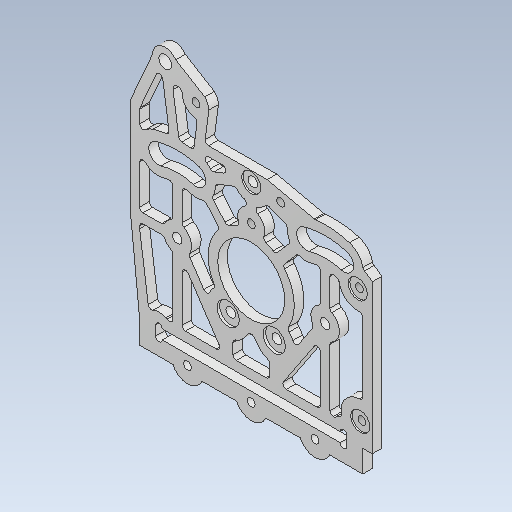
# Autodesk Inventor part: 中間フレーム内側
Saved by Autodesk Inventor 2020.2 (Build 242310000, 310)
## iProperties
Created: 2020-03-13
Part Number: 中間フレーム内側
Material: アルミニウム 2014-T4
Document SubType Name: Modeling
Designer: aoyam
Density: 2.8 g/cm^3
Appearance: サテン
Mass: 22.5667 g
Surface Area: 94.6631 cm^2
Volume: 8.05954 cm^3
Author: aoyam
Autodesk Inventor part; units mm, degrees
ref_plane "YZ Plane" through (0, 0, 0) normal (1, 0, 0) x (0, 1, 0)
ref_plane "XZ Plane" through (0, 0, 0) normal (0, 1, 0) x (-1, 0, 0)
ref_plane "XY Plane" through (0, 0, 0) normal (0, 0, 1) x (1, 0, 0)
sketch "スケッチ1" plane through (0, 0, 0) normal (0, 0, 1) x (1, 0, 0)
  circle A0 centre (0, 15.5) radius 1.25
  circle A1 centre (0, -15.5) radius 1.5
  line L0 (0, 0) -> (100, 0)
  line L1 (0, 15.5) -> (0, -15.5)
  circle A2 centre (23.2, 20.8573) radius 1.5
  circle A3 centre (23.2, 0) radius 1.5
  line L2 (23.2, 20.8573) -> (23.2, 0)
  line L3 (23.2, 0) -> (90.6993, -20)
  line L4 (23.2, 0) -> (29.1254, 19.9979)
  line L5 (23.2, 0) -> (17.2746, 19.9979)
  arc A4 (29.1254, 19.9979) -> (17.2746, 19.9979) centre (23.2, 0) ccw construction
  arc A5 (29.9847, 22.8983) -> (16.4153, 22.8983) centre (23.2, 0) ccw
  arc A6 (28.266, 17.0975) -> (18.134, 17.0975) centre (23.2, 0) ccw
  arc A7 (28.266, 17.0975) -> (29.9847, 22.8983) centre (29.1254, 19.9979) ccw
  arc A8 (16.4153, 22.8983) -> (18.134, 17.0975) centre (17.2746, 19.9979) ccw
  circle A9 centre (0, 0) radius 10.5
  circle A10 centre (0, 0) radius 14.1421
  circle A11 centre (0, 15.5) radius 4.5
  circle A12 centre (0, -15.5) radius 4.5
  line L6 (0, 30) -> (38, 30)
  line L7 (38, 30) -> (38, -28)
  line L8 (38, -28) -> (0, -28)
  line L9 (0, -28) -> (0, 30)
  circle A13 centre (-23.2, 0) radius 1.5
  arc A14 (-16.4153, 22.8983) -> (-29.9847, 22.8983) centre (-23.2, 0) ccw
  arc A15 (-18.134, 17.0975) -> (-28.266, 17.0975) centre (-23.2, 0) ccw
  arc A16 (-29.9847, 22.8983) -> (-28.266, 17.0975) centre (-29.1254, 19.9979) ccw
  arc A17 (-18.134, 17.0975) -> (-16.4153, 22.8983) centre (-17.2746, 19.9979) ccw
  line L10 (0, 30) -> (-38, 30)
  line L11 (-38, 30) -> (-38, -28)
  line L12 (-38, -28) -> (0, -28)
  line L13 (-38, -27) -> (38, -27)
  line L14 (-30, -27) -> (30, -27)
  line L15 (30, -27) -> (30, -30)
  line L16 (30, -30) -> (-30, -30)
  line L17 (-30, -30) -> (-30, -27)
  line L18 (0, -27) -> (0, -33)
  circle A18 centre (0, -33) radius 1.25
  circle A19 centre (-20, -33) radius 1.25
  circle A20 centre (20, -33) radius 1.25
  circle A21 centre (-20, -33) radius 5
  circle A22 centre (0, -33) radius 5
  circle A23 centre (20, -33) radius 5
  line L19 (35, -22) -> (-35, -22)
  line L20 (-35, -22) -> (-35, -35)
  line L21 (-35, -35) -> (35, -35)
  line L22 (35, -35) -> (35, -22)
  circle A24 centre (-28.95, -27) radius 1.05
  line L23 (-30, -27) -> (-28.95, -27)
  line L24 (-12.3917, -28.5) -> (-10.5848, -28.5)
  circle A25 centre (-28.95, -30) radius 1.05
  circle A26 centre (28.95, -27) radius 1.05
  circle A27 centre (28.95, -30) radius 1.05
  line L25 (30, -27) -> (30, -30)
  line L26 (-30, -27) -> (-30, -30)
  circle A28 centre (-27, 46) radius 2
  circle A29 centre (-27, 46) radius 4
  line L27 (-38, 30) -> (-31, 46)
  line L28 (-23.4377, 47.8194) -> (-19, 30)
  circle A30 centre (-17.3043, 39.7432) radius 4
  circle A31 centre (-17.3043, 39.7432) radius 1.25
  line L29 (-23.6785, 48.2289) -> (-14.5834, 42.6752)
  line L30 (-13.3043, 39.7432) -> (-14.5834, 30)
  line L31 (27.4137, -1.5794) -> (34.5946, 17.4704)
  arc A32 (34.5946, 17.4704) -> (30.837, 25.7747) centre (29.1254, 19.9979) ccw
  arc A33 (30.837, 25.7747) -> (23.2, 26.8823) centre (23.2, 0) ccw
  line L32 (23.2, 26.8823) -> (-8.2253, 30.1221)
  arc A34 (-8.2253, 30.1221) -> (-10.295, 30.1221) centre (-9.2601, 26) ccw
  line L33 (-10.295, 30.1221) -> (-23.2, 26.8823)
  arc A35 (-23.2, 26.8823) -> (-30.837, 25.7747) centre (-23.2, 0) ccw
  arc A36 (-30.837, 25.7747) -> (-34.7286, 17.7833) centre (-29.1254, 19.9979) ccw
  line L34 (-34.7286, 17.7833) -> (-27.7, 0)
  arc A37 (-27.7, 0) -> (-25.9762, -3.5416) centre (-23.2, 0) ccw
  line L35 (-25.9762, -3.5416) -> (-10.0045, -16.0614)
  arc A38 (-10.0045, -16.0614) -> (-7.2283, -17.0198) centre (-7.2283, -12.5198) ccw
  line L36 (-7.2283, -17.0198) -> (7.2283, -17.0198)
  arc A39 (7.2283, -17.0198) -> (10.0045, -16.0614) centre (7.2283, -12.5198) ccw
  line L37 (10.0045, -16.0614) -> (25.9762, -3.5416)
  arc A40 (25.9762, -3.5416) -> (27.4137, -1.5794) centre (23.2, 0) ccw
  circle A41 centre (-7.2283, -12.5198) radius 1.5
  circle A42 centre (23.2, 0) radius 1.5
  circle A43 centre (-23.2, 0) radius 1.5
  circle A44 centre (7.2283, -12.5198) radius 1.5
  circle A45 centre (-9.2601, 26) radius 1.25
  arc A46 (28.266, 17.0975) -> (29.9847, 22.8983) centre (29.1254, 19.9979) ccw
  arc A47 (28.266, 17.0975) -> (18.134, 17.0975) centre (23.2, 0) ccw
  arc A48 (16.4153, 22.8983) -> (18.134, 17.0975) centre (17.2746, 19.9979) ccw
  arc A49 (29.9847, 22.8983) -> (16.4153, 22.8983) centre (23.2, 0) ccw
  arc A50 (-29.9847, 22.8983) -> (-28.266, 17.0975) centre (-29.1254, 19.9979) ccw
  arc A51 (-16.4153, 22.8983) -> (-29.9847, 22.8983) centre (-23.2, 0) ccw
  arc A52 (-18.134, 17.0975) -> (-16.4153, 22.8983) centre (-17.2746, 19.9979) ccw
  arc A53 (-18.134, 17.0975) -> (-28.266, 17.0975) centre (-23.2, 0) ccw
  circle A54 centre (9.2601, 26) radius 1.25
  point P0 (0, 0)
  point P1 (24.7, 0)
  point P2 (38, 0)
  point P3 (38, -4.3852)
  point P4 (24.6382, -0.4261)
  point P5 (0.6086, 14.129)
  point P6 (-0.6086, 14.129)
  point P7 (30, -27)
  point P8 (-35, -28)
  point P9 (-24.5826, -35)
  point P10 (-15.4174, -35)
  point P11 (-4.5826, -35)
  point P12 (4.5826, -35)
  point P13 (15.4174, -35)
  point P14 (24.5826, -35)
  point P15 (35, -28)
  point P16 (-27.9, -30)
  point P17 (-30, -30)
  point P18 (-30, -28.4849)
  point P19 (-27.9, -27)
  point P20 (27.9, -27)
  point P21 (30, -27)
  point P22 (30, -30)
  point P23 (27.9, -30)
  point P24 (-30, -30)
  point P25 (-30, -28)
  point P26 (-29.2702, -28)
  point P27 (29.2702, -28)
  point P28 (30, -28)
  point P29 (29.9846, -28.5)
  point P30 (28.5305, -28.5)
  point P31 (-29.9846, -28.5)
  point P32 (-28.5305, -28.5)
  point P33 (0, -30)
  point P34 (0, -28)
  point P35 (0, -27)
  point P36 (-27.9, -27)
  point P37 (-30, -30)
  point P38 (0, -27)
  point P39 (30, -28)
  point P40 (28.6298, -28)
  point P41 (27.9, -27)
  point P42 (0, -28)
  point P43 (30, -27)
  point P44 (15, 30)
  point P45 (-23.0005, 46.0638)
  dimension "d90" = 2.1
  dimension "d0" = 100
  dimension "d1" = 15.5
  dimension "d2" = 15.5
  dimension "d3" = 3
  dimension "d4" = 2.5
  dimension "d5" = 31
  dimension "d10" = 23.2
  dimension "d12" = 20.8573
  dimension "d13" = 70.4
  dimension "d14" = 90
  dimension "d15" = 20.8573
  dimension "d16" = 20
  dimension "d17" = 6.05
  dimension "d18" = 3
  dimension "d24" = 21
  dimension "d27" = 3.6421
  dimension "d28" = 30
  dimension "d29" = 28
  dimension "d30" = 38
  dimension "d70" = 1
  dimension "d71" = 60
  dimension "d72" = 3
  dimension "d73" = 30
  dimension "d76" = 6
  dimension "d77" = 2.5
  dimension "d80" = 20
  dimension "d85" = 10
  dimension "d86" = 10
  dimension "d87" = 10
  dimension "d88" = 5
  dimension "d93" = 1.5
  dimension "d97" = 4
  dimension "d98" = 8
  dimension "d102" = 8
  dimension "d103" = 2.5
  dimension "d262" = 73
  dimension "d264" = 3
  constraints: 76 end point, 58 point on circle, 52 centre point, 18 symmetric about line, 7 coincident, 7 point on line, 7 vertical, 6 horizontal, 6 parallel, 5 tangent, 4 perpendicular, 3 midpoint, 26 other
  measures "d0" distance of L0.start L0.end
  measures "d1" distance of L1.start L0.start
  measures "d2" distance of L1.end L0.start
  measures "d3" diameter of A1
  measures "d4" diameter of A0
  measures "d5" distance of L1.start L1.end
  measures "d10" distance of L0.start L2.end
  measures "d12" distance of L2.start L2.end
  measures "d13" distance of L2.end L3.end
  measures "d14" angle of L3 L4
  measures "d15" distance of L2.end L4.end
  measures "d16" distance from line of L0 L3.end
  measures "d17" diameter of A8
  measures "d18" diameter of A3
  measures "d24" diameter of A9
  measures "d27" radial gap between concentric circles of A9 A10
  measures "d28" distance from line of L6.end L0
  measures "d29" distance from line of L7.end L0
  measures "d30" distance between parallel lines of L9 L7
  measures "d70" distance between parallel lines of L8 L13
  measures "d71" distance of L15.end L16.end
  measures "d72" distance of L14.end L15.end
  measures "d73" distance between parallel lines of L9 L15
  measures "d76" distance of L18.start L18.end
  measures "d77" diameter of A18
  measures "d80" distance of A18.centre A19.centre
  measures "d85" diameter of A21
  measures "d86" diameter of A22
  measures "d87" diameter of A23
  measures "d88" distance between parallel lines of L13 L19
  measures "d93" distance between parallel lines of L24 L14
  measures "d97" diameter of A28
  measures "d98" diameter of A29
  measures "d102" diameter of A30
  measures "d103" diameter of A31
  measures "d262" distance from line of L14 A28.centre
  measures "d264" distance from line of L17 A28.centre
extrude "押し出し1" add sketch "スケッチ1" along normal blind 3 contours A0 L9 A11 A10 L1 | A0 L1 A10 A11 L9 | L9 L32 A33 A32 L31 L0 A3 L4 A7 A5 A8 L5 A10 A11 | A11 A10 A41 A12 L36 A38 L35 A37 L34 A36 A35 L33 L10 L32 L9 | A10 A11 L1 | L1 A11 A10 | A11 L1 A9 A12 A10 A41 | L32 L10 L9 | L9 L6 L7 L0 L31 A32 A33 L32 | A11 A10 L0 A9 L1 | A41 A10 | A10 A41 | A10 A44 A12 L1 A9 L0 | L0 A3 L3 L31 A40 L37 A39 L36 A12 A10 A44 | L33 A35 A36 L34 A37 L35 A38 L36 A12 L9 L19 L20 L13 L11 L10 | A44 A10 | A10 A44 | A12 L1 A1 A10 | A10 A1 L9 L36 A12 | L7 L3 L31 L0 | L10 L28 A30 L30 | A12 A10 A1 L1 | L5 A6 L2 A3 | A3 L0 L31 L3 | A10 L1 L9 A1 | A1 L1 A10 | L36 L9 A12 | L7 L13 L22 L19 L9 A12 L36 A39 L37 A40 L31 L3 | L10 L27 A29 L28 | A30 L29 L30 | A1 A10 L1 | A12 L36 L9 A1 A10 | L2 A6 L4 A3 | L9 L1 A10 A1 | L9 L36 A12 | L7 L8 L22 L13 | L28 A29 L29 A30 | L19 L22 L13 A26 L9 | L9 L13 A24 L20 L19 | L22 L8 L15 L13 | L13 L20 L12 L11 | A29 L28 | L28 A29 | L22 L21 A23 L16 A27 L15 L8 | L13 L17 L12 L20 | L12 L17 A25 L16 A21 L21 L20 | L16 A22 L21 | L16 A23 L21 A22 | A22 L21 A21 L16 | L21 A23 L16 | A23 L21 | A21 L21 L16 | L21 A22 | L21 A21 | A45
sketch "スケッチ8" plane through (0, 0, 3) normal (0, 0, 1) x (1, 0, 0)
  line L0 (0, 0) -> (0, 13.1)
  line L1 (26.2, 7.3075) -> (26.2, 0)
  line L2 (-139.7061, -70) -> (112.711, -70)
  line L3 (-139.7061, -20) -> (112.711, -20)
  line L4 (-139.7231, -25) -> (112.694, -25)
  circle A0 centre (0, 0) radius 20.05
  circle A1 centre (14.8447, 16.629) radius 2.05
  circle A2 centre (14.8447, 16.629) radius 14
  circle A3 centre (19.3878, -11) radius 2.05
  circle A4 centre (19.3878, -11) radius 14
  circle A5 centre (0, 0) radius 9.1
  line L5 (0, 0) -> (-93.6, 0)
  circle A6 centre (-93.6, 0) radius 25.1
  circle A7 centre (-52.6656, -10.2575) radius 17.1
  circle A8 centre (-23.2, 0) radius 14.1
  circle A9 centre (23.2, 0) radius 14.1
  circle A10 centre (52.6656, -10.2575) radius 17.1
  line L6 (0, 0) -> (93.6, 0)
  circle A11 centre (93.6, 0) radius 25.1
  dimension "d53" = 7.3075
  dimension "d54" = 70
  dimension "d55" = 50
  dimension "d56" = 45
  dimension "d57" = 4.1
  dimension "d58" = 28
  dimension "d59" = 4.1
  dimension "d60" = 28
  dimension "d61" = 22.291
  dimension "d62" = 22.291
  dimension "d63" = 40.1
  dimension "d64" = 18.2
  dimension "d65" = 93.6
  dimension "d66" = 50.2
  dimension "d67" = 34.2
  dimension "d68" = 28.2
  dimension "d69" = 70.4
  constraints: 14 end point, 12 centre point, 7 coincident, 5 tangent, 4 symmetric about line, 3 horizontal, 3 point on line, 2 parallel, 1 vertical, 3 other
  measures "d53" distance of L1.start L1.end
  measures "d54" distance from line of L2 point (0, 0)
  measures "d55" distance between parallel lines of L2 L3
  measures "d56" distance between parallel lines of L2 L4
  measures "d57" diameter of A1
  measures "d58" diameter of A2
  measures "d59" diameter of A3
  measures "d60" diameter of A4
  measures "d61" distance of A1.centre point (0, 0)
  measures "d62" distance of A3.centre point (0, 0)
  measures "d63" diameter of A0
  measures "d64" diameter of A5
  measures "d65" distance of L0.start L5.end
  measures "d66" diameter of A6
  measures "d67" diameter of A7
  measures "d68" diameter of A8
  measures "d69" distance of L5.end A8.centre
sketch "スケッチ3" plane through (0, 0, 0) normal (0, 0, -1) x (-1, 0, 0)
  arc A0 (1.6057, 5.7812) -> (-1.6057, 5.7812) centre (0, 0) ccw
  line L0 (-1.5, -5.8095) -> (-1.5, -12.9019)
  arc A1 (-1.5, -12.9019) -> (1.5, -12.9019) centre (0, -15.5) ccw
  line L1 (1.5, -12.9019) -> (1.5, -5.8095)
  arc A2 (1.5, -5.8095) -> (4.2038, 4.2812) centre (0, 0) ccw
  circle A3 centre (0, -15.5) radius 1.5
  circle A4 centre (0, 0) radius 4
  arc A5 (-4.2038, 4.2812) -> (-1.5, -5.8095) centre (0, 0) ccw
  line L2 (4.2038, 4.2812) -> (6.406, 8.0955)
  circle A6 centre (7.2283, 12.5198) radius 3
  line L3 (3.8079, 9.5955) -> (1.6057, 5.7812)
  line L4 (-1.6057, 5.7812) -> (-3.8079, 9.5955)
  circle A7 centre (-7.2283, 12.5198) radius 3
  line L5 (-6.406, 8.0955) -> (-4.2038, 4.2812)
  arc A8 (6.406, 8.0955) -> (3.8079, 9.5955) centre (7.2283, 12.5198) ccw
  arc A9 (-3.8079, 9.5955) -> (-6.406, 8.0955) centre (-7.2283, 12.5198) ccw
  line L6 (0, 0) -> (-9.4783, 0)
  circle A10 centre (7.2283, -12.5198) radius 3
  circle A11 centre (-7.2283, -12.5198) radius 3
  circle A12 centre (-7.2283, -12.5198) radius 1.5
  circle A13 centre (7.2283, -12.5198) radius 1.5
  point P0 (0, 0)
  point P1 (0, 0)
  dimension "d36" = 3
  dimension "d37" = 3
  constraints: 14 centre point, 14 end point, 12 point on circle, 2 coincident, 2 symmetric about line, 1 horizontal, 4 other
  measures "d36" diameter of A12
  measures "d37" diameter of A13
extrude "押し出し3" cut sketch "スケッチ3" against normal blind 10 contours A12 | A13
sketch "スケッチ2" plane through (0, 0, 3) normal (0, 0, 1) x (1, 0, 0)
  circle A0 centre (0, 15.5) radius 1.25 projected
  circle A1 centre (0, 15.5) radius 3.5
  circle A2 centre (7.2283, -12.5198) radius 1.5 projected
  circle A3 centre (-7.2283, -12.5198) radius 1.5 projected
  circle A4 centre (-7.2283, -12.5198) radius 3.5
  circle A5 centre (7.2283, -12.5198) radius 3.5
  point P0 (0, 0)
  dimension "d33" = 7
  dimension "d40" = 7
  dimension "d41" = 7
  constraints: 3 centre point, 3 coincident
  measures "d33" diameter of A1
  measures "d40" diameter of A4
  measures "d41" diameter of A5
extrude "押し出し2" cut sketch "スケッチ2" against normal blind 0.8 contours A4 | A5
sketch "スケッチ4" plane through (0, 0, 0) normal (0, 0, -1) x (-1, 0, 0)
  circle A0 centre (7.2283, -12.5198) radius 1.5 projected
  circle A1 centre (-7.2283, -12.5198) radius 1.5 projected
  circle A2 centre (-23.2, 0) radius 1.5 projected
  arc A3 (-18.134, 17.0975) -> (-28.266, 17.0975) centre (-23.2, 0) ccw projected
  arc A4 (-29.9847, 22.8983) -> (-28.266, 17.0975) centre (-29.1254, 19.9979) ccw projected
  arc A5 (-16.4153, 22.8983) -> (-29.9847, 22.8983) centre (-23.2, 0) ccw projected
  arc A6 (-18.134, 17.0975) -> (-16.4153, 22.8983) centre (-17.2746, 19.9979) ccw projected
  circle A7 centre (0, 15.5) radius 1.25 projected
  circle A8 centre (0, 0) radius 10.5 projected
  circle A9 centre (23.2, 0) radius 1.5 projected
  arc A10 (28.266, 17.0975) -> (18.134, 17.0975) centre (23.2, 0) ccw projected
  arc A11 (16.4153, 22.8983) -> (18.134, 17.0975) centre (17.2746, 19.9979) ccw projected
  arc A12 (29.9847, 22.8983) -> (16.4153, 22.8983) centre (23.2, 0) ccw projected
  arc A13 (28.266, 17.0975) -> (29.9847, 22.8983) centre (29.1254, 19.9979) ccw projected
  line L0 (-38, -28) -> (-38, 30) projected
  line L1 (-35, -28) -> (-38, -28) projected
  line L2 (38, 30) -> (38, -28) projected
  line L3 (-38, 30) -> (14.5834, 30) projected
  line L4 (-35, -35) -> (-35, -28) projected
  line L5 (-24.5826, -35) -> (-35, -35) projected
  arc A14 (-24.5826, -35) -> (-15.4174, -35) centre (-20, -33) ccw projected
  line L6 (-4.5826, -35) -> (-15.4174, -35) projected
  arc A15 (-4.5826, -35) -> (4.5826, -35) centre (0, -33) ccw projected
  line L7 (15.4174, -35) -> (4.5826, -35) projected
  arc A16 (15.4174, -35) -> (24.5826, -35) centre (20, -33) ccw projected
  line L8 (35, -35) -> (24.5826, -35) projected
  line L9 (35, -28) -> (35, -35) projected
  line L10 (38, -28) -> (35, -28) projected
  line L11 (31, 46) -> (38, 30) projected
  arc A17 (31, 46) -> (23.6785, 48.2289) centre (27, 46) ccw projected
  line L12 (14.5834, 42.6752) -> (23.6785, 48.2289) projected
  arc A18 (14.5834, 42.6752) -> (13.3043, 39.7432) centre (17.3043, 39.7432) ccw projected
  line L13 (14.5834, 30) -> (13.3043, 39.7432) projected
sketch "スケッチ5" plane through (0, 0, 3) normal (0, 0, 1) x (1, 0, 0)
  line L0 (-28.272, 25.2385) -> (-28.272, -21.075)
  line L1 (-28.272, -21.075) -> (37.1454, -21.075)
  line L2 (37.1454, -21.075) -> (37.1454, 25.2385)
  line L3 (37.1454, 25.2385) -> (-28.272, 25.2385)
  circle A0 centre (20.8127, 11.3014) radius 1.3
  circle A1 centre (8.8768, 21.9566) radius 1.3
  circle A2 centre (14.8447, 16.629) radius 2.05
  circle A3 centre (33.4387, 14.579) radius 1.25
  circle A4 centre (15.4401, -17.9581) radius 1.3
  circle A5 centre (23.3356, -4.0419) radius 1.3
  circle A6 centre (19.3878, -11) radius 2.05
  circle A7 centre (0, 26.6903) radius 1.5
  circle A8 centre (34.2063, -21.075) radius 1.25
  point P0 (0, 0)
  point P1 (0, 0)
  dimension "d270" = 2.5
  dimension "d271" = 2.5
  constraints: 9 centre point, 8 end point, 2 horizontal, 2 vertical, 1 point on line, 22 other
  measures "d270" diameter of A3
  measures "d271" diameter of A8
extrude "押し出し4" cut sketch "スケッチ5" against normal blind 10 contours A7 L3 | L3 A7 | A8 L1 | L1 A8 | A3
sketch "スケッチ6" plane through (0, 0, 3) normal (0, 0, 1) x (1, 0, 0)
  circle A0 centre (0, 26.6903) radius 1.5 projected
  circle A1 centre (34.2063, -21.075) radius 1.25 projected
  circle A2 centre (33.4387, 14.579) radius 1.25 projected
  circle A3 centre (0, 26.6903) radius 3
  circle A4 centre (34.2063, -21.075) radius 3
  circle A5 centre (33.4387, 14.579) radius 3
  point P0 (0, 0)
  dimension "d44" = 6
  dimension "d45" = 6
  dimension "d46" = 6
  constraints: 3 centre point, 3 coincident
  measures "d44" diameter of A3
  measures "d45" diameter of A4
  measures "d46" diameter of A5
extrude "押し出し5" cut sketch "スケッチ6" against normal blind 0.5
fillet "フィレット1" radius 6 2 edges at (38, 30, 1.5) (-38, 30, 1.5)
sketch "スケッチ9" plane through (0, 0, 3) normal (0, 0, 1) x (1, 0, 0)
  circle A0 centre (0, 26.6903) radius 1.5 projected
  circle A1 centre (33.4387, 14.579) radius 1.25 projected
  circle A2 centre (0, 0) radius 10.5 projected
  circle A3 centre (34.2063, -21.075) radius 1.25 projected
  circle A4 centre (23.2, 0) radius 1.5 projected
thread "ねじ1" size "M3x0.5" class "6H" standard "ANSI Metric M Profile" full length
sketch "ダンパ" plane through (0, 0, 0) normal (0, 0, -1) x (-1, 0, 0)
  circle A0 centre (27.1179, 46.6808) radius 5.0025 projected
  circle A1 centre (17.3043, 39.7432) radius 1.25 projected
  line L0 (17.3043, 39.7432) -> (-58.0131, 55.7524)
  line L1 (0, 0) -> (-70, 0)
  circle A2 centre (-58.0131, 55.7524) radius 1.25
  dimension "d104" = 77
  dimension "d105" = 12
  dimension "d106" = 2.5
  constraints: 4 end point, 1 centre point, 1 coincident
  measures "d104" distance of L0.start L0.end
  measures "d105" angle of L1 L0
  measures "d106" diameter of A2
sketch "スケッチ11" plane through (0, 0, 3) normal (0, 0, 1) x (1, 0, 0)
  arc A0 (-38, 28.7449) -> (-37.4969, 31.1498) centre (-32, 28.7449) ccw projected
  line L0 (-38, 28.7449) -> (-38, -28) projected
  line L1 (38, -28) -> (38, 24) projected
  arc A1 (32, 30) -> (38, 24) centre (32, 24) ccw projected
  line L2 (32, 30) -> (-14.5834, 30) projected
  line L3 (-14.5834, 30) -> (-13.3043, 39.7432) projected
  arc A2 (-13.3043, 39.7432) -> (-14.5834, 42.6752) centre (-17.3043, 39.7432) ccw projected
  line L4 (-14.5834, 42.6752) -> (-23.6785, 48.2289) projected
  arc A3 (-23.6785, 48.2289) -> (-31, 46) centre (-27, 46) ccw projected
  line L5 (-31, 46) -> (-37.4969, 31.1498) projected
  circle A4 centre (33.4387, 14.579) radius 3 projected
  circle A5 centre (34.2063, -21.075) radius 3 projected
  circle A6 centre (0, 26.6903) radius 3 projected
  circle A7 centre (7.2283, -12.5198) radius 3.5 projected
  circle A8 centre (-7.2283, -12.5198) radius 3.5 projected
  circle A9 centre (23.2, 0) radius 1.5 projected
  circle A10 centre (0, 15.5) radius 1.25 projected
  arc A11 (27.9, -27) -> (30, -27) centre (28.95, -27) ccw projected
  line L6 (30, -27) -> (30, -30) projected
  arc A12 (30, -30) -> (27.9, -30) centre (28.95, -30) ccw projected
  line L7 (27.9, -30) -> (-27.9, -30) projected
  arc A13 (-27.9, -30) -> (-30, -30) centre (-28.95, -30) ccw projected
  line L8 (-30, -30) -> (-30, -27) projected
  arc A14 (-30, -27) -> (-27.9, -27) centre (-28.95, -27) ccw projected
  line L9 (-27.9, -27) -> (27.9, -27) projected
  arc A15 (-18.134, 17.0975) -> (-28.266, 17.0975) centre (-23.2, 0) ccw projected
  arc A16 (-28.266, 17.0975) -> (-29.9847, 22.8983) centre (-29.1254, 19.9979) ccw projected
  arc A17 (-29.9847, 22.8983) -> (-16.4153, 22.8983) centre (-23.2, 0) ccw projected
  arc A18 (-16.4153, 22.8983) -> (-18.134, 17.0975) centre (-17.2746, 19.9979) ccw projected
  circle A19 centre (-23.2, 0) radius 1.5 projected
  circle A20 centre (0, 0) radius 10.5 projected
  arc A21 (16.4153, 22.8983) -> (29.9847, 22.8983) centre (23.2, 0) ccw projected
  arc A22 (29.9847, 22.8983) -> (28.266, 17.0975) centre (29.1254, 19.9979) ccw projected
  arc A23 (28.266, 17.0975) -> (18.134, 17.0975) centre (23.2, 0) ccw projected
  arc A24 (18.134, 17.0975) -> (16.4153, 22.8983) centre (17.2746, 19.9979) ccw projected
  circle A25 centre (-27, 46) radius 2 projected
  circle A26 centre (-17.3043, 39.7432) radius 1.25 projected
  line L10 (-35, -28) -> (-35, 29.3725)
  line L11 (-35, 29.3725) -> (-27.3163, 46.9351)
  line L12 (-27.3163, 46.9351) -> (-16.2712, 40.1908)
  line L13 (-16.2712, 40.1908) -> (-18.003, 27)
  line L14 (-18.003, 27) -> (35, 27)
  line L15 (35, 27) -> (35, -28)
  arc A27 (33, -27) -> (26.2292, -24) centre (28.95, -27) ccw
  line L16 (33, -27) -> (33, -30)
  arc A28 (26.2292, -33) -> (33, -30) centre (28.95, -30) ccw
  line L17 (26.2292, -33) -> (-26.2292, -33)
  arc A29 (-33, -30) -> (-26.2292, -33) centre (-28.95, -30) ccw
  line L18 (-33, -30) -> (-33, -27)
  arc A30 (-26.2292, -24) -> (-33, -27) centre (-28.95, -27) ccw
  line L19 (-26.2292, -24) -> (26.2292, -24)
  circle A31 centre (-27, 46) radius 5
  circle A32 centre (-17.3043, 39.7432) radius 4.25
  arc A33 (-30.837, 25.7747) -> (-27.4137, 14.2211) centre (-29.1254, 19.9979) ccw
  arc A34 (-18.9863, 14.2211) -> (-27.4137, 14.2211) centre (-23.2, 0) ccw
  arc A35 (-18.9863, 14.2211) -> (-15.563, 25.7747) centre (-17.2746, 19.9979) ccw
  arc A36 (-15.563, 25.7747) -> (-30.837, 25.7747) centre (-23.2, 0) ccw
  circle A37 centre (-23.2, 0) radius 4.5
  circle A38 centre (-7.2283, -12.5198) radius 6.5
  circle A39 centre (0, 0) radius 13.5
  circle A40 centre (7.2283, -12.5198) radius 6.5
  circle A41 centre (0, 15.5) radius 4.25
  circle A42 centre (0, 26.6903) radius 6
  arc A43 (27.4137, 14.2211) -> (18.9863, 14.2211) centre (23.2, 0) ccw
  arc A44 (27.4137, 14.2211) -> (30.837, 25.7747) centre (29.1254, 19.9979) ccw
  arc A45 (30.837, 25.7747) -> (15.563, 25.7747) centre (23.2, 0) ccw
  arc A46 (15.563, 25.7747) -> (18.9863, 14.2211) centre (17.2746, 19.9979) ccw
  circle A47 centre (33.4387, 14.579) radius 6
  circle A48 centre (23.2, 0) radius 4.5
  circle A49 centre (34.2063, -21.075) radius 6
  line L20 (-34.9021, 0) -> (-23.2, 0) construction
  line L21 (-34.9021, -1.5) -> (-23.2, -1.5)
  line L22 (-23.2, 1.5) -> (-34.9021, 1.5)
  arc A50 (-34.9021, 1.5) -> (-34.9021, -1.5) centre (-34.9021, 0) ccw
  arc A51 (-23.2, -1.5) -> (-23.2, 1.5) centre (-23.2, 0) ccw
  line L23 (-23.2, 0) -> (-23.2, -24) construction
  line L24 (-24.7, 0) -> (-24.7, -24)
  line L25 (-21.7, -24) -> (-21.7, 0)
  arc A52 (-21.7, 0) -> (-24.7, 0) centre (-23.2, 0) ccw
  arc A53 (-24.7, -24) -> (-21.7, -24) centre (-23.2, -24) ccw
  line L26 (-23.2, 0) -> (-23.2, 20.579) construction
  line L27 (-21.7, 0) -> (-21.7, 20.579)
  line L28 (-24.7, 20.579) -> (-24.7, 0)
  arc A54 (-24.7, 0) -> (-21.7, 0) centre (-23.2, 0) ccw
  arc A55 (-21.7, 20.579) -> (-24.7, 20.579) centre (-23.2, 20.579) ccw
  line L29 (-17.2746, 19.9979) -> (0, 0) construction
  line L30 (-18.4098, 19.0173) -> (-1.1351, -0.9806)
  line L31 (1.1351, 0.9806) -> (-16.1395, 20.9784)
  arc A56 (-16.1395, 20.9784) -> (-18.4098, 19.0173) centre (-17.2746, 19.9979) ccw
  arc A57 (-1.1351, -0.9806) -> (1.1351, 0.9806) centre (0, 0) ccw
  line L32 (-23.2, 20.579) -> (-27, 46) construction
  line L33 (-21.7165, 20.8007) -> (-25.5165, 46.2218)
  line L34 (-28.4835, 45.7782) -> (-24.6835, 20.3572)
  arc A58 (-24.6835, 20.3572) -> (-21.7165, 20.8007) centre (-23.2, 20.579) ccw
  arc A59 (-25.5165, 46.2218) -> (-28.4835, 45.7782) centre (-27, 46) ccw
  line L35 (-17.2746, 19.9979) -> (0, 26.6903) construction
  line L36 (-16.7328, 18.5992) -> (0.5419, 25.2916)
  line L37 (-0.5419, 28.089) -> (-17.8165, 21.3966)
  arc A60 (-17.8165, 21.3966) -> (-16.7328, 18.5992) centre (-17.2746, 19.9979) ccw
  arc A61 (0.5419, 25.2916) -> (-0.5419, 28.089) centre (0, 26.6903) ccw
  line L38 (0, 26.6903) -> (17.2746, 19.9979) construction
  line L39 (-0.5419, 25.2916) -> (16.7328, 18.5992)
  line L40 (17.8165, 21.3966) -> (0.5419, 28.089)
  arc A62 (0.5419, 28.089) -> (-0.5419, 25.2916) centre (0, 26.6903) ccw
  arc A63 (16.7328, 18.5992) -> (17.8165, 21.3966) centre (17.2746, 19.9979) ccw
  line L41 (0, 0) -> (17.2746, 19.9979) construction
  line L42 (1.1351, -0.9806) -> (18.4098, 19.0173)
  line L43 (16.1395, 20.9784) -> (-1.1351, 0.9806)
  arc A64 (-1.1351, 0.9806) -> (1.1351, -0.9806) centre (0, 0) ccw
  arc A65 (18.4098, 19.0173) -> (16.1395, 20.9784) centre (17.2746, 19.9979) ccw
  line L44 (-7.2283, -12.5198) -> (-7.2283, -24) construction
  line L45 (-8.7283, -12.5198) -> (-8.7283, -24)
  line L46 (-5.7283, -24) -> (-5.7283, -12.5198)
  arc A66 (-5.7283, -12.5198) -> (-8.7283, -12.5198) centre (-7.2283, -12.5198) ccw
  arc A67 (-8.7283, -24) -> (-5.7283, -24) centre (-7.2283, -24) ccw
  circle A68 centre (-28.8146, 40.8909) radius 1.05
  circle A69 centre (-33.95, 25.1727) radius 1.05
  circle A70 centre (-33.95, 14.8231) radius 1.05
  circle A71 centre (-23.0525, 39.8846) radius 1.5
  circle A72 centre (-18.9817, 27.6119) radius 1.05
  circle A73 centre (-13.45, 25.95) radius 1.05
  circle A74 centre (-8.9697, 25.95) radius 1.05
  circle A75 centre (-25.75, -22.95) radius 1.05
  circle A76 centre (-10.1996, 20.0042) radius 1.05
  circle A77 centre (0, -15.9479) radius 1.5
  line L47 (-23.2, 0) -> (-7.2283, -24) construction
  line L48 (-24.4488, -0.831) -> (-8.4771, -24.831)
  line L49 (-5.9795, -23.169) -> (-21.9512, 0.831)
  arc A78 (-21.9512, 0.831) -> (-24.4488, -0.831) centre (-23.2, 0) ccw
  arc A79 (-8.4771, -24.831) -> (-5.9795, -23.169) centre (-7.2283, -24) ccw
  line L50 (0, 15.5) -> (0, 10.5)
  line L51 (35, -28) -> (35, 29.3725)
  line L52 (34.9021, -1.5) -> (23.2, -1.5)
  line L53 (23.2, 1.5) -> (34.9021, 1.5)
  line L54 (24.7, 0) -> (24.7, -24)
  line L55 (21.7, -24) -> (21.7, 0)
  line L56 (21.7, 0) -> (21.7, 20.579)
  line L57 (24.7, 20.579) -> (24.7, 0)
  line L58 (8.7283, -12.5198) -> (8.7283, -24)
  line L59 (5.7283, -24) -> (5.7283, -12.5198)
  circle A80 centre (13.45, 25.95) radius 1.05
  circle A81 centre (8.9697, 25.95) radius 1.05
  circle A82 centre (33.95, -25.995) radius 1.05
  circle A83 centre (25.75, -22.95) radius 1.05
  circle A84 centre (10.1996, 20.0042) radius 1.05
  line L60 (24.4488, -0.831) -> (8.4771, -24.831)
  line L61 (5.9795, -23.169) -> (21.9512, 0.831)
  circle A85 centre (-20.65, -8.4345) radius 1.05
  circle A86 centre (20.65, -8.4345) radius 1.05
  arc A87 (-37.4969, 31.1498) -> (-38, 28.7449) centre (-32, 28.7449) ccw projected
  line L62 (-38, 28.7449) -> (-38, -28) projected
  line L63 (-38, -28) -> (-35, -28) projected
  line L64 (-35, -28) -> (-35, -35) projected
  line L65 (-35, -35) -> (-24.5826, -35) projected
  arc A88 (-24.5826, -35) -> (-15.4174, -35) centre (-20, -33) ccw projected
  line L66 (-15.4174, -35) -> (-4.5826, -35) projected
  arc A89 (-4.5826, -35) -> (4.5826, -35) centre (0, -33) ccw projected
  line L67 (4.5826, -35) -> (15.4174, -35) projected
  arc A90 (15.4174, -35) -> (24.5826, -35) centre (20, -33) ccw projected
  line L68 (24.5826, -35) -> (35, -35) projected
  line L69 (35, -35) -> (35, -28) projected
  line L70 (35, -28) -> (38, -28) projected
  line L71 (38, -28) -> (38, 24) projected
  arc A91 (38, 24) -> (32, 30) centre (32, 24) ccw projected
  line L72 (32, 30) -> (-14.5834, 30) projected
  line L73 (-14.5834, 30) -> (-13.3043, 39.7432) projected
  arc A92 (-13.3043, 39.7432) -> (-14.5834, 42.6752) centre (-17.3043, 39.7432) ccw projected
  line L74 (-14.5834, 42.6752) -> (-23.6785, 48.2289) projected
  arc A93 (-23.6785, 48.2289) -> (-31, 46) centre (-27, 46) ccw projected
  line L75 (-31, 46) -> (-37.4969, 31.1498) projected
  circle A94 centre (33.4387, 14.579) radius 3 projected
  circle A95 centre (34.2063, -21.075) radius 3 projected
  circle A96 centre (0, 26.6903) radius 3 projected
  circle A97 centre (7.2283, -12.5198) radius 3.5 projected
  circle A98 centre (-7.2283, -12.5198) radius 3.5 projected
  circle A99 centre (23.2, 0) radius 1.5 projected
  circle A100 centre (0, 15.5) radius 1.25 projected
  arc A101 (30, -27) -> (27.9, -27) centre (28.95, -27) ccw projected
  line L76 (30, -27) -> (30, -30) projected
  arc A102 (27.9, -30) -> (30, -30) centre (28.95, -30) ccw projected
  line L77 (27.9, -30) -> (-27.9, -30) projected
  arc A103 (-30, -30) -> (-27.9, -30) centre (-28.95, -30) ccw projected
  line L78 (-30, -30) -> (-30, -27) projected
  arc A104 (-27.9, -27) -> (-30, -27) centre (-28.95, -27) ccw projected
  line L79 (-27.9, -27) -> (27.9, -27) projected
  arc A105 (-18.134, 17.0975) -> (-28.266, 17.0975) centre (-23.2, 0) ccw projected
  arc A106 (-29.9847, 22.8983) -> (-28.266, 17.0975) centre (-29.1254, 19.9979) ccw projected
  arc A107 (-16.4153, 22.8983) -> (-29.9847, 22.8983) centre (-23.2, 0) ccw projected
  arc A108 (-18.134, 17.0975) -> (-16.4153, 22.8983) centre (-17.2746, 19.9979) ccw projected
  circle A109 centre (-23.2, 0) radius 1.5 projected
  circle A110 centre (0, 0) radius 10.5 projected
  circle A111 centre (20, -33) radius 1.25 projected
  circle A112 centre (-20, -33) radius 1.25 projected
  circle A113 centre (0, -33) radius 1.25 projected
  arc A114 (29.9847, 22.8983) -> (16.4153, 22.8983) centre (23.2, 0) ccw projected
  arc A115 (28.266, 17.0975) -> (29.9847, 22.8983) centre (29.1254, 19.9979) ccw projected
  arc A116 (28.266, 17.0975) -> (18.134, 17.0975) centre (23.2, 0) ccw projected
  arc A117 (16.4153, 22.8983) -> (18.134, 17.0975) centre (17.2746, 19.9979) ccw projected
  circle A118 centre (-27, 46) radius 2 projected
  circle A119 centre (-17.3043, 39.7432) radius 1.25 projected
  circle A120 centre (-2.5803, 20.1295) radius 1.05
  circle A121 centre (2.5803, 20.1295) radius 1.05
  line L80 (-25.75, -22.95) -> (-35, 0) construction
  line L81 (-24.5906, -22.4827) -> (-33.8406, 0.4673)
  line L82 (-36.1594, -0.4673) -> (-26.9094, -23.4173)
  arc A122 (-26.9094, -23.4173) -> (-24.5906, -22.4827) centre (-25.75, -22.95) ccw
  arc A123 (-33.8406, 0.4673) -> (-36.1594, -0.4673) centre (-35, 0) ccw
  line L83 (-35.8943, -1.125) -> (-38, 0.7321)
  line L84 (-32.085, -24.4359) -> (-35, -28)
  line L85 (-38, 0.7321) -> (-35, -28)
  line L86 (-32.085, -24.4359) -> (-35, -3.3438)
  line L87 (5.0046, 30) -> (19.9931, 26.6903)
  point P0 (-29.0511, 0)
  point P1 (-23.2, -12)
  point P2 (-23.2, 10.2895)
  point P3 (-8.6373, 9.9989)
  point P4 (-25.1, 33.2895)
  point P5 (-8.6373, 23.3441)
  point P6 (8.6373, 23.3441)
  point P7 (8.6373, 9.9989)
  point P8 (-7.2283, -18.2599)
  point P9 (-15.2142, -12)
  point P10 (24.7, -4.2426)
  point P11 (24.7, -22.95)
  point P12 (25.75, -24)
  point P13 (28.5145, -22.9735)
  point P14 (35, -15.1277)
  point P15 (35, 8.7857)
  point P16 (27.45, 14.2105)
  point P17 (24.7, 14.7562)
  point P18 (24.7, 4.2426)
  point P19 (13.6656, -11.6194)
  point P20 (19.6007, -2.701)
  point P21 (21.7, 4.2426)
  point P22 (21.7, 14.7562)
  point P23 (14.5952, 14.6015)
  point P24 (9.9054, 9.1724)
  point P25 (11.2713, -7.4302)
  point P26 (19.7759, -7.8528)
  point P27 (9.0301, -24)
  point P28 (21.7, -8.4345)
  point P29 (5.7283, -18.8443)
  point P30 (1.3553, -15.3051)
  point P31 (-1.3553, -15.3051)
  point P32 (-5.7283, -18.8443)
  point P33 (-21.7, -8.4345)
  point P34 (-9.0301, -24)
  point P35 (-19.7759, -7.8528)
  point P36 (-19.6007, -2.701)
  point P37 (-13.6656, -11.6194)
  point P38 (-11.2713, -7.4302)
  point P39 (-9.9054, 9.1724)
  point P40 (-14.5952, 14.6015)
  point P41 (-21.7, 14.7562)
  point P42 (-21.7, 4.2426)
  point P43 (8.5904, 24.9709)
  point P44 (12.3753, 23.5046)
  point P45 (14.0176, 25.0666)
  point P46 (13.45, 27)
  point P47 (8.9697, 27)
  point P48 (-11.2496, 20.0032)
  point P49 (-12.325, 16.5626)
  point P50 (-7.6352, 11.1335)
  point P51 (-3.4702, 13.0464)
  point P52 (3.4702, 13.0464)
  point P53 (7.6352, 11.1335)
  point P54 (12.325, 16.5626)
  point P55 (11.2496, 20.0032)
  point P56 (10.579, 20.9833)
  point P57 (4.8753, 23.1929)
  point P58 (-4.8753, 23.1929)
  point P59 (-10.579, 20.9833)
  point P60 (-8.9697, 27)
  point P61 (-13.45, 27)
  point P62 (-14.0176, 25.0666)
  point P63 (-12.3753, 23.5046)
  point P64 (-8.5904, 24.9709)
  point P65 (-21.553, 39.8477)
  point P66 (-24.536, 39.6628)
  point P67 (-22.6246, 26.8761)
  point P68 (-19.1403, 26.574)
  point P69 (-17.9406, 27.4752)
  point P70 (-16.8852, 35.5139)
  point P71 (-33.234, 24.4047)
  point P72 (-25.6423, 26.7711)
  point P73 (-27.7761, 41.0461)
  point P74 (-29.7766, 41.3117)
  point P75 (-35, 25.1727)
  point P76 (-35, 14.8231)
  point P77 (-35, 1.4968)
  point P78 (-27.4426, 1.5)
  point P79 (-24.7, 4.2426)
  point P80 (-24.7, 14.7562)
  point P81 (-33.234, 15.5911)
  point P82 (-24.7, -22.95)
  point P83 (-24.7, -4.2426)
  point P84 (-27.4426, -1.5)
  point P85 (-35, -1.4968)
  point P86 (-25.75, -24)
  point P87 (5.0046, 30)
  point P88 (5.959, 25.9903)
  point P89 (14.0176, 25.0667)
  point P90 (35, 21.3355)
  point P91 (26.8038, 27)
  point P92 (35.1092, 20.7011)
  point P93 (38, 18.7436)
  point P94 (38, 24)
  point P95 (-2.196, 21.1066)
  point P96 (-11.2496, 20.0032)
  point P97 (-2.0691, 19.2123)
  point P98 (2.0691, 19.2123)
  point P99 (11.2496, 20.0042)
  point P100 (2.196, 21.1066)
  point P101 (-30.375, -11.475)
  point P102 (-33.0477, -1.5)
  point P103 (-24.7, -22.2114)
  point P104 (-26.8553, -23.5338)
  point P105 (-38, 0.7321)
  point P106 (-35, -3.3438)
  point P107 (-26.7157, -23.6221)
  point P108 (-25.1384, -23.8035)
  point P109 (-38, 0.7321)
  point P110 (5.0046, 30)
  dimension "d215" = 3
  dimension "d216" = 3
  dimension "d217" = 3
  dimension "d218" = 3
  dimension "d219" = 3
  dimension "d220" = 3
  dimension "d221" = 3
  dimension "d222" = 3
  dimension "d223" = 3
  dimension "d224" = 3
  dimension "d225" = 3
  dimension "d226" = 3
  dimension "d227" = 3
  dimension "d228" = 3
  dimension "d229" = 3
  dimension "d230" = 3
  dimension "d231" = 3
  dimension "d232" = 3
  dimension "d233" = 1.5
  dimension "d234" = 3
  dimension "d235" = 3
  dimension "d236" = 3
  dimension "d237" = 3
  dimension "d238" = 3
  dimension "d239" = 2.1
  dimension "d240" = 2.1
  dimension "d241" = 2.1
  dimension "d242" = 3
  dimension "d243" = 2.1
  dimension "d244" = 2.1
  dimension "d245" = 2.1
  dimension "d247" = 2.1
  dimension "d248" = 2.1
  dimension "d249" = 3
  dimension "d250" = 3
  dimension "d251" = 2.1
  dimension "d252" = 2.1
  dimension "d265" = 2.1
  dimension "d266" = 2.1
  dimension "d267" = 2.5
  constraints: 142 end point, 89 centre point, 71 point on circle, 70 tangent, 25 symmetric about line, 11 midpoint, 11 parallel, 10 point on line, 1 vertical alignment, 29 other
  measures "d215" distance between parallel lines of L5 L11
  measures "d216" distance between parallel lines of L9 L19
  measures "d217" radial gap between concentric circles of A25 A31
  measures "d218" radial gap between concentric circles of A26 A32
  measures "d219" radial gap between concentric circles of A17 A36
  measures "d220" radial gap between concentric circles of A19 A37
  measures "d221" radial gap between concentric circles of A8 A38
  measures "d223" radial gap between concentric circles of A7 A40
  measures "d224" radial gap between concentric circles of A10 A41
  measures "d225" radius of A6
  measures "d226" radial gap between concentric circles of A23 A43
  measures "d227" radial gap between concentric circles of A4 A47
  measures "d228" radial gap between concentric circles of A9 A48
  measures "d229" radial gap between concentric circles of A5 A49
  measures "d230" diameter of A51
  measures "d231" diameter of A53
  measures "d232" diameter of A55
  measures "d233" radius of A57
  measures "d234" diameter of A59
  measures "d235" diameter of A61
  measures "d236" diameter of A63
  measures "d237" diameter of A65
  measures "d238" diameter of A67
  measures "d239" diameter of A68
  measures "d240" diameter of A69
  measures "d241" diameter of A70
  measures "d242" diameter of A71
  measures "d243" diameter of A72
  measures "d244" diameter of A73
  measures "d245" diameter of A74
  measures "d247" diameter of A75
  measures "d248" diameter of A76
  measures "d249" diameter of A77
  measures "d250" diameter of A79
  measures "d251" diameter of A85
  measures "d252" diameter of A86
  measures "d265" diameter of A120
  measures "d266" diameter of A121
  measures "d267" diameter of A123
extrude "押し出し6" cut sketch "スケッチ11" against normal blind 3 contours L10 L11 A0 L34 A36 A33 A69 | A69 | L85 A17 L0 | A17 L85 L63 L0 | A68 A31 | A31 A68 | L11 A68 L34 A0 | A0 L34 A36 | L10 A70 A33 A34 L28 A37 L22 A50 | A50 L21 L81 L24 A75 A17 A30 A122 L82 L10 | L82 A122 A30 A17 L86 | A70 | A71 | L33 A71 A32 L13 A72 A36 | A17 A30 L86 | A72 | L21 A37 L24 L81 | A34 A35 L30 A39 A38 L49 A37 L27 | A73 L14 A74 L37 A35 | A73 | A75 A17 | L2 A1 L14 L87 | A74 | L36 A42 A120 A41 A17 A76 | A76 A17 | L25 A17 L48 L19 | A35 A76 A17 A41 A39 L31 | A91 L51 L14 A1 | L14 A1 A45 L87 | A17 A76 | A85 L48 A17 L25 | A85 | L14 L15 A44 A45 A1 | A91 A1 A21 A44 L15 L51 | A120 | L1 A21 A1 | A42 L39 A84 A21 A41 A121 | A121 | L46 A38 A77 A40 L59 L19 | A84 A21 | A77 | A84 A21 | A84 A46 L43 A39 A41 A21 | L60 A21 L55 L19 | L15 A49 A27 A21 A83 L54 A48 L57 A43 A44 A47 | L60 A86 L55 A21 | A27 L19 A83 A21 | A39 L42 A46 A43 L56 A48 L61 A40 | A86 | A83 A21 | A21 A83 picked at (-25.7663, -23.1259)
fillet "フィレット2" radius 1.05 53 edges at (-35, -1.4968, 1.5) (-27.4426, -1.5, 1.5) (-24.7, -4.2426, 1.5) (-35, 1.4968, 1.5) (-27.4426, 1.5, 1.5) (-24.7, 4.2426, 1.5) (-24.7, 14.7562, 1.5) (-25.6423, 26.7711, 1.5) (-35, 29.3725, 1.5) (-22.6246, 26.8761, 1.5) (-16.8852, 35.5139, 1.5) (-14.5952, 14.6015, 1.5) (-21.7, 14.7562, 1.5) (-21.7, 4.2426, 1.5) (-19.6007, -2.701, 1.5) (-13.6656, -11.6194, 1.5) (-11.2713, -7.4302, 1.5) (-9.9054, 9.1724, 1.5) (-9.0301, -24, 1.5) (-21.7, -24, 1.5) (-5.7283, -24, 1.5) (-5.7283, -18.8443, 1.5) (5.7283, -24, 1.5) (5.7283, -18.8443, 1.5) (-12.3753, 23.5046, 1.5) (-7.6352, 11.1335, 1.5) (-3.4702, 13.0464, 1.5) (-12.325, 16.5626, 1.5) (3.4702, 13.0464, 1.5) (-4.8753, 23.1929, 1.5) (4.8753, 23.1929, 1.5) (7.6352, 11.1335, 1.5) (12.325, 16.5626, 1.5) (21.7, 4.2426, 1.5) (19.6007, -2.701, 1.5) (14.5952, 14.6015, 1.5) (21.7, 14.7562, 1.5) (9.9054, 9.1724, 1.5) (11.2713, -7.4302, 1.5) (13.6656, -11.6194, 1.5) (9.0301, -24, 1.5) (21.7, -24, 1.5) (28.5145, -22.9735, 1.5) (35, -15.1277, 1.5) (27.45, 14.2105, 1.5) (35, 8.7857, 1.5) (24.7, 14.7562, 1.5) (24.7, -4.2426, 1.5) (24.7, 4.2426, 1.5) (-26.7157, -23.6221, 1.5) (-32.085, -24.4359, 1.5) (-35, -28, 1.5) (19.9931, 26.6903, 1.5)
fillet "フィレット3" radius 1.05 2 edges at (35.1092, 20.7011, 1.5) (-14.5834, 30, 1.5)
thread "ねじ2" size "M3x0.5" class "6H" standard "ANSI Metric M Profile" full length
thread "ねじ3" size "M3x0.5" class "6H" standard "ANSI Metric M Profile" full length
thread "ねじ4" size "M3x0.5" class "6H" standard "ANSI Metric M Profile" length 44.8
thread "ねじ5" size "M3x0.5" class "6H" standard "ANSI Metric M Profile" length 44.8
equation "\"d15\" = d12"
